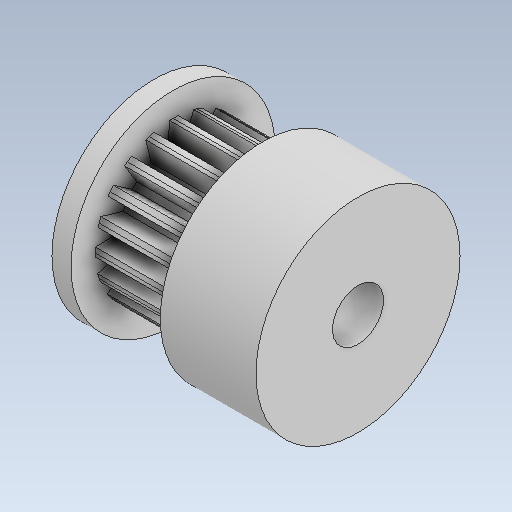
# Autodesk Inventor part: gear_20
Saved by Autodesk Inventor 2020 (Build 240168000, 168)
## iProperties
Created: 2024-02-19
Part Number: gear_20
Material: Типовые
Document SubType Name: Modeling
Designer: 4s
Density: 1 g/cm^3
Appearance: По умолчанию
Author: 4s
Autodesk Inventor part; units mm, degrees
ref_plane "YZ Plane" through (0, 0, 0) normal (1, 0, 0) x (0, 1, 0)
ref_plane "XZ Plane" through (0, 0, 0) normal (0, 1, 0) x (-1, 0, 0)
ref_plane "XY Plane" through (0, 0, 0) normal (0, 0, 1) x (1, 0, 0)
sketch "Эскиз1" plane through (0, 0, 0) normal (1, 0, 0) x (0, 1, 0)
  circle A0 centre (0, 0) radius 6.1
  dimension "d0" = 12.2
  constraints: 1 centre point, 1 coincident
  measures "d0" diameter of A0
extrude "Выдавливание1" add sketch "Эскиз1" along normal blind 7
sketch "Эскиз2" plane through (7, 0, 0) normal (1, 0, 0) x (0, 0, -1)
  circle A0 centre (0, 0) radius 8
  dimension "d3" = 16
  constraints: 1 centre point, 1 coincident
  measures "d3" diameter of A0
extrude "Выдавливание2" add sketch "Эскиз2" along normal blind 7.5
sketch "Эскиз3" plane through (0, 0, 0) normal (-1, 0, 0) x (0, 0, 1)
  circle A0 centre (0, 0) radius 8
  circle A1 centre (0, 0) radius 6.1 construction
  circle A2 centre (0, 0) radius 6.1 construction
  circle A3 centre (0, 0) radius 8 construction
  circle A4 centre (0, 0) radius 8 construction
  circle A5 centre (0, 0) radius 4.3 construction
  line L0 (0, 0) -> (0, 6.1) construction
  line L1 (0, 0) -> (-1.885, 5.8014) construction
  line L2 (0, 6.1) -> (-0.4001, 6.0869)
  line L3 (-0.4001, 6.0869) -> (-0.4458, 4.2768)
  line L4 (-0.4458, 4.2768) -> (-0.9294, 4.1984)
  line L5 (-0.9294, 4.1984) -> (-1.6222, 5.8803)
  line L6 (-1.6222, 5.8803) -> (-1.885, 5.8014)
  line L7 (-1.885, 5.8014) -> (-2.2615, 5.6653)
  line L8 (-2.2615, 5.6653) -> (-1.7456, 3.9297)
  line L9 (-1.7456, 3.9297) -> (-2.1813, 3.7057)
  line L10 (-2.1813, 3.7057) -> (-3.36, 5.0912)
  line L11 (-3.36, 5.0912) -> (-3.5855, 4.935)
  line L12 (-3.5855, 4.935) -> (-3.9015, 4.6892)
  line L13 (-3.9015, 4.6892) -> (-2.8746, 3.198)
  line L14 (-2.8746, 3.198) -> (-3.2196, 2.8502)
  line L15 (-3.2196, 2.8502) -> (-4.7688, 3.8038)
  line L16 (-4.7688, 3.8038) -> (-4.935, 3.5855)
  line L17 (-4.935, 3.5855) -> (-5.1596, 3.2541)
  line L18 (-5.1596, 3.2541) -> (-3.7221, 2.1532)
  line L19 (-3.7221, 2.1532) -> (-3.9428, 1.7158)
  line L20 (-3.9428, 1.7158) -> (-5.7108, 2.144)
  line L21 (-5.7108, 2.144) -> (-5.8014, 1.885)
  line L22 (-5.8014, 1.885) -> (-5.9126, 1.5004)
  line L23 (-5.9126, 1.5004) -> (-4.2053, 0.8976)
  line L24 (-4.2053, 0.8976) -> (-4.2801, 0.4134)
  line L25 (-4.2801, 0.4134) -> (-6.0938, 0.2743)
  line L26 (-6.0938, 0.2743) -> (-6.1, 0)
  line L27 (-6.1, 0) -> (-6.0869, -0.4001)
  line L28 (-6.0869, -0.4001) -> (-4.2768, -0.4458)
  line L29 (-4.2768, -0.4458) -> (-4.1984, -0.9294)
  line L30 (-4.1984, -0.9294) -> (-5.8803, -1.6222)
  line L31 (-5.8803, -1.6222) -> (-5.8014, -1.885)
  line L32 (-5.8014, -1.885) -> (-5.6653, -2.2615)
  line L33 (-5.6653, -2.2615) -> (-3.9297, -1.7456)
  line L34 (-3.9297, -1.7456) -> (-3.7057, -2.1813)
  line L35 (-3.7057, -2.1813) -> (-5.0912, -3.36)
  line L36 (-5.0912, -3.36) -> (-4.935, -3.5855)
  line L37 (-4.935, -3.5855) -> (-4.6892, -3.9015)
  line L38 (-4.6892, -3.9015) -> (-3.198, -2.8746)
  line L39 (-3.198, -2.8746) -> (-2.8502, -3.2196)
  line L40 (-2.8502, -3.2196) -> (-3.8038, -4.7688)
  line L41 (-3.8038, -4.7688) -> (-3.5855, -4.935)
  line L42 (-3.5855, -4.935) -> (-3.2541, -5.1596)
  line L43 (-3.2541, -5.1596) -> (-2.1532, -3.7221)
  line L44 (-2.1532, -3.7221) -> (-1.7158, -3.9428)
  line L45 (-1.7158, -3.9428) -> (-2.144, -5.7108)
  line L46 (-2.144, -5.7108) -> (-1.885, -5.8014)
  line L47 (-1.885, -5.8014) -> (-1.5004, -5.9126)
  line L48 (-1.5004, -5.9126) -> (-0.8976, -4.2053)
  line L49 (-0.8976, -4.2053) -> (-0.4134, -4.2801)
  line L50 (-0.4134, -4.2801) -> (-0.2743, -6.0938)
  line L51 (-0.2743, -6.0938) -> (0, -6.1)
  line L52 (0, -6.1) -> (0.4001, -6.0869)
  line L53 (0.4001, -6.0869) -> (0.4458, -4.2768)
  line L54 (0.4458, -4.2768) -> (0.9294, -4.1984)
  line L55 (0.9294, -4.1984) -> (1.6222, -5.8803)
  line L56 (1.6222, -5.8803) -> (1.885, -5.8014)
  line L57 (1.885, -5.8014) -> (2.2615, -5.6653)
  line L58 (2.2615, -5.6653) -> (1.7456, -3.9297)
  line L59 (1.7456, -3.9297) -> (2.1813, -3.7057)
  line L60 (2.1813, -3.7057) -> (3.36, -5.0912)
  line L61 (3.36, -5.0912) -> (3.5855, -4.935)
  line L62 (3.5855, -4.935) -> (3.9015, -4.6892)
  line L63 (3.9015, -4.6892) -> (2.8746, -3.198)
  line L64 (2.8746, -3.198) -> (3.2196, -2.8502)
  line L65 (3.2196, -2.8502) -> (4.7688, -3.8038)
  line L66 (4.7688, -3.8038) -> (4.935, -3.5855)
  line L67 (4.935, -3.5855) -> (5.1596, -3.2541)
  line L68 (5.1596, -3.2541) -> (3.7221, -2.1532)
  line L69 (3.7221, -2.1532) -> (3.9428, -1.7158)
  line L70 (3.9428, -1.7158) -> (5.7108, -2.144)
  line L71 (5.7108, -2.144) -> (5.8014, -1.885)
  line L72 (5.8014, -1.885) -> (5.9126, -1.5004)
  line L73 (5.9126, -1.5004) -> (4.2053, -0.8976)
  line L74 (4.2053, -0.8976) -> (4.2801, -0.4134)
  line L75 (4.2801, -0.4134) -> (6.0938, -0.2743)
  line L76 (6.0938, -0.2743) -> (6.1, 0)
  line L77 (6.1, 0) -> (6.0869, 0.4001)
  line L78 (6.0869, 0.4001) -> (4.2768, 0.4458)
  line L79 (4.2768, 0.4458) -> (4.1984, 0.9294)
  line L80 (4.1984, 0.9294) -> (5.8803, 1.6222)
  line L81 (5.8803, 1.6222) -> (5.8014, 1.885)
  line L82 (5.8014, 1.885) -> (5.6653, 2.2615)
  line L83 (5.6653, 2.2615) -> (3.9297, 1.7456)
  line L84 (3.9297, 1.7456) -> (3.7057, 2.1813)
  line L85 (3.7057, 2.1813) -> (5.0912, 3.36)
  line L86 (5.0912, 3.36) -> (4.935, 3.5855)
  line L87 (4.935, 3.5855) -> (4.6892, 3.9015)
  line L88 (4.6892, 3.9015) -> (3.198, 2.8746)
  line L89 (3.198, 2.8746) -> (2.8502, 3.2196)
  line L90 (2.8502, 3.2196) -> (3.8038, 4.7688)
  line L91 (3.8038, 4.7688) -> (3.5855, 4.935)
  line L92 (3.5855, 4.935) -> (3.2541, 5.1596)
  line L93 (3.2541, 5.1596) -> (2.1532, 3.7221)
  line L94 (2.1532, 3.7221) -> (1.7158, 3.9428)
  line L95 (1.7158, 3.9428) -> (2.144, 5.7108)
  line L96 (2.144, 5.7108) -> (1.885, 5.8014)
  line L97 (1.885, 5.8014) -> (1.5004, 5.9126)
  line L98 (1.5004, 5.9126) -> (0.8976, 4.2053)
  line L99 (0.8976, 4.2053) -> (0.4134, 4.2801)
  line L100 (0.4134, 4.2801) -> (0.2743, 6.0938)
  line L101 (0.2743, 6.0938) -> (0, 6.1)
  circle A6 centre (0, 0) radius 6.909
  dimension "d6" = 16
  dimension "d12" = 8.6
  dimension "d13" = 18
  dimension "d16" = 360
  constraints: 204 end point, 6 point on circle, 3 centre point, 3 coincident, 1 vertical, 221 other
  measures "d6" diameter of A0
  measures "d12" diameter of A5
  measures "d13" angle of L0 L1
extrude "Выдавливание3" add sketch "Эскиз3" along normal blind 1.5 contours A0 | L101 L100 L99 L98 L97 L96 L95 L94 L93 L92 L91 L90 L89 L88 L87 L86 L85 L84 L83 L82 L81 L80 L79 L78 L77 L76 L75 L74 L73 L72 L71 L70 L69 L68 L67 L66 L65 L64 L63 L62 L61 L60 L59 L58 L57 L56 L55 L54 L53 L52 L51 L50 L49 L48 L47 L46 L45 L44 L43 L42 L41 L40 L39 L38 L37 L36 L35 L34 L33 L32 L31 L30 L29 L28 L27 L26 L25 L24 L23 L22 L21 L20 L19 L18 L17 L16 L15 L14 L13 L12 L11 L10 L9 L8 L7 L6 L5 L4 L3 L2 | A6
sketch "Эскиз4" plane through (14.5, 0, 0) normal (1, 0, 0) x (0, 0, -1)
  circle A0 centre (0, 0) radius 2
  dimension "d9" = 4
  constraints: 1 centre point, 1 coincident
  measures "d9" diameter of A0
extrude "Выдавливание4" cut sketch "Эскиз4" against normal up to surface (16 mm away)
extrude "Выдавливание5" cut sketch "Эскиз3" against normal up to surface (7 mm away) contours A6
